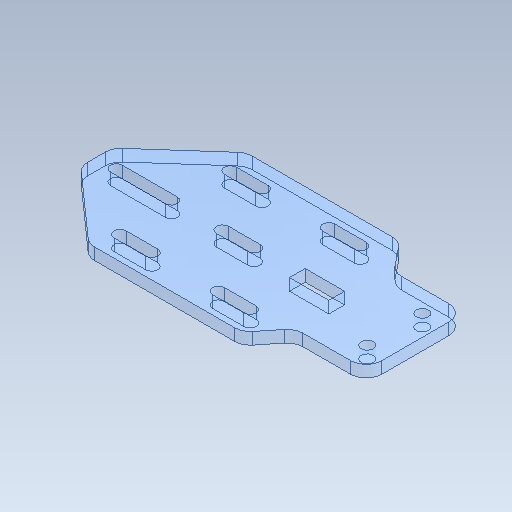
# Autodesk Inventor part: pulsador_monta_servo
Saved by Autodesk Inventor 2022 (Build 260153000, 153)
## iProperties
Created: 2022-11-16
Part Number: pulsador_monta_servo
Material: Generic
Document SubType Name: Modeling
Designer: ferna
Density: 1 g/cm^3
Appearance: Blue - Glazing
Author: ferna
Autodesk Inventor part; units mm, degrees
ref_plane "YZ Plane" through (0, 0, 0) normal (1, 0, 0) x (0, 1, 0)
ref_plane "XZ Plane" through (0, 0, 0) normal (0, 1, 0) x (-1, 0, 0)
ref_plane "XY Plane" through (0, 0, 0) normal (0, 0, 1) x (1, 0, 0)
sketch3d "3D Sketch1"
sketch "Sketch8" plane through (0, 0, 0) normal (0, 1, 0) x (-1, 0, 0)
  arc A0 (-533.9727, 129.2939) -> (-533.9727, 72.7061) centre (-524, 101) ccw projected
  arc A1 (-533.9727, 129.2939) -> (-540.6211, 148.1565) centre (-537.2969, 138.7252) ccw projected
  arc A2 (-540.6211, 148.1565) -> (-540.6211, 53.8435) centre (-524, 101) ccw projected
  arc A3 (-540.6211, 53.8435) -> (-533.9727, 72.7061) centre (-537.2969, 63.2748) ccw projected
  circle A4 centre (-537.2969, 63.2748) radius 3 projected
  circle A5 centre (-556.6482, 77.8001) radius 2.9994 projected
  circle A6 centre (-564, 101) radius 3 projected
  circle A7 centre (-556.6482, 124.1094) radius 2.9994 projected
  circle A8 centre (-537.2969, 138.7252) radius 3 projected
  line L0 (-531, 98.5) -> (-531, 115.5) projected
  line L1 (-451.3425, 101.8066) -> (-466.8633, 88.0104) projected
  arc A9 (-451.3425, 101.8066) -> (-450, 104.7963) centre (-454, 104.7963) ccw projected
  line L2 (-450, 109.2037) -> (-450, 104.7963) projected
  arc A10 (-450, 109.2037) -> (-451.3425, 112.1934) centre (-454, 109.2037) ccw projected
  line L3 (-466.8633, 125.9896) -> (-451.3425, 112.1934) projected
  arc A11 (-466.8633, 125.9896) -> (-469.5208, 127) centre (-469.5208, 123) ccw projected
  line L4 (-505.0775, 127) -> (-469.5208, 127) projected
  arc A12 (-505.0775, 127) -> (-508.201, 125.4988) centre (-505.0775, 123) ccw projected
  line L5 (-511.799, 121.0012) -> (-508.201, 125.4988) projected
  arc A13 (-514.9225, 119.5) -> (-511.799, 121.0012) centre (-514.9225, 123.5) ccw projected
  line L6 (-527, 119.5) -> (-514.9225, 119.5) projected
  arc A14 (-527, 119.5) -> (-531, 115.5) centre (-527, 115.5) ccw projected
  arc A15 (-531, 98.5) -> (-527, 94.5) centre (-527, 98.5) ccw projected
  line L7 (-514.9225, 94.5) -> (-527, 94.5) projected
  arc A16 (-511.799, 92.9988) -> (-514.9225, 94.5) centre (-514.9225, 90.5) ccw projected
  line L8 (-508.201, 88.5012) -> (-511.799, 92.9988) projected
  arc A17 (-508.201, 88.5012) -> (-505.0775, 87) centre (-505.0775, 91) ccw projected
  line L9 (-469.5208, 87) -> (-505.0775, 87) projected
  line L10 (-478, 91.45) -> (-470, 91.45) projected
  arc A18 (-470, 91.45) -> (-470, 94.55) centre (-470, 93) ccw projected
  line L11 (-470, 94.55) -> (-478, 94.55) projected
  arc A19 (-478, 94.55) -> (-478, 91.45) centre (-478, 93) ccw projected
  arc A20 (-495, 91.45) -> (-495, 94.55) centre (-495, 93) ccw projected
  line L12 (-503, 91.45) -> (-495, 91.45) projected
  arc A21 (-503, 94.55) -> (-503, 91.45) centre (-503, 93) ccw projected
  line L13 (-495, 94.55) -> (-503, 94.55) projected
  line L14 (-455, 105.5) -> (-469, 105.5) projected
  arc A22 (-455, 105.5) -> (-455, 108.5) centre (-455, 107) ccw projected
  line L15 (-469, 108.5) -> (-455, 108.5) projected
  arc A23 (-469, 108.5) -> (-469, 105.5) centre (-469, 107) ccw projected
  arc A24 (-482, 105.45) -> (-482, 108.55) centre (-482, 107) ccw projected
  line L16 (-490, 105.45) -> (-482, 105.45) projected
  arc A25 (-490, 108.55) -> (-490, 105.45) centre (-490, 107) ccw projected
  line L17 (-482, 108.55) -> (-490, 108.55) projected
  line L18 (-501, 109) -> (-501, 105) projected
  line L19 (-501, 105) -> (-511, 105) projected
  line L20 (-511, 105) -> (-511, 109) projected
  line L21 (-511, 109) -> (-501, 109) projected
  circle A26 centre (-525.75, 100) radius 1.55 projected
  circle A27 centre (-525.75, 114) radius 1.55 projected
  arc A28 (-503, 122.55) -> (-503, 119.45) centre (-503, 121) ccw projected
  line L22 (-503, 122.55) -> (-495, 122.55) projected
  arc A29 (-495, 119.45) -> (-495, 122.55) centre (-495, 121) ccw projected
  line L23 (-495, 119.45) -> (-503, 119.45) projected
  arc A30 (-478, 122.55) -> (-478, 119.45) centre (-478, 121) ccw projected
  line L24 (-478, 122.55) -> (-470, 122.55) projected
  arc A31 (-470, 119.45) -> (-470, 122.55) centre (-470, 121) ccw projected
  line L25 (-470, 119.45) -> (-478, 119.45) projected
  arc A32 (-469.5208, 87) -> (-466.8633, 88.0104) centre (-469.5208, 91) ccw projected
  point P0 (0, 0)
extrude "Extrusion1" add sketch "Sketch8" along normal blind 3 contours L0 A14 L6 A13 L5 A12 L4 A11 L3 A10 L2 A9 L1 A32 L9 A17 L8 A16 L7 A15
body "Solid1"
